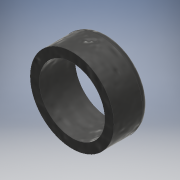
# Autodesk Inventor part: Tires
Saved by Autodesk Inventor 2018 (Build 220112000, 112)
## iProperties
Created: 2017-09-24
Part Number: Tires
Material: Generic
Document SubType Name: Modeling
Designer: Yikealo
Density: 1 g/cm^3
Appearance: Default
Author: Yikealo
Autodesk Inventor part; units mm, degrees
ref_plane "YZ Plane" through (0, 0, 0) normal (1, 0, 0) x (0, 1, 0)
ref_plane "XZ Plane" through (0, 0, 0) normal (0, 1, 0) x (-1, 0, 0)
ref_plane "XY Plane" through (0, 0, 0) normal (0, 0, 1) x (1, 0, 0)
sketch "Sketch2" plane through (0, 0, 0) normal (0, 1, 0) x (-1, 0, 0)
  circle A0 centre (0, 0) radius 11.5
  dimension "d2" = 23
  constraints: 1 centre point, 1 coincident
  measures "d2" diameter of A0
extrude "Extrusion1" add sketch "Sketch2" along normal blind 9.8
sketch "Sketch3" plane through (0, 9.8, 0) normal (0, 1, 0) x (1, 0, 0)
  circle A0 centre (0, 0) radius 9
  dimension "d5" = 18
  constraints: 1 centre point, 1 coincident
  measures "d5" diameter of A0
extrude "Extrusion2" cut sketch "Sketch3" against normal through all
fillet "Fillet1" radius 2 1 edges at (11.5, 9.8, 0)
body "Solid1"
